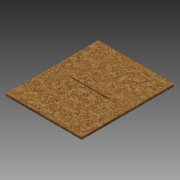
# Autodesk Inventor part: gora
Saved by Autodesk Inventor 2013 (Build 170138000, 138)
## iProperties
Created: 2014-04-26
Part Number: gora
Material: Generic
Document SubType Name: Modeling
Designer: Masta
Density: 1 g/cm^3
Author: Masta
Autodesk Inventor part; units mm, degrees
ref_plane "YZ Plane" through (0, 0, 0) normal (1, 0, 0) x (0, 1, 0)
ref_plane "XZ Plane" through (0, 0, 0) normal (0, 1, 0) x (-1, 0, 0)
ref_plane "XY Plane" through (0, 0, 0) normal (0, 0, 1) x (1, 0, 0)
sketch "Sketch1" plane through (0, 0, 0) normal (0, 0, 1) x (1, 0, 0)
  line L0 (-300, -366) -> (300, -366)
  line L1 (300, -366) -> (300, 366)
  line L2 (300, 366) -> (-300, 366)
  line L3 (-300, 366) -> (-300, -366)
  line L4 (-300, -366) -> (300, 366) construction
  line L5 (300, -366) -> (-300, 366) construction
  line L6 (150, 10) -> (-150, 10)
  line L7 (-150, 10) -> (-150, 0)
  line L8 (-150, 0) -> (150, 0)
  line L9 (150, 0) -> (150, 10)
  line L10 (150, 10) -> (-150, 0) construction
  line L11 (-150, 10) -> (150, 0) construction
  line L12 (0, 0) -> (0, 5) construction
  dimension "d0" = 600
  dimension "d1" = 732
  dimension "d4" = 300
  dimension "d5" = 10
  dimension "d6" = 5
  constraints: 26 end point, 5 parallel, 4 midpoint, 2 horizontal, 2 perpendicular
  measures "d0" distance of L2.end L1.end
  measures "d1" distance of L1.end L0.end
  measures "d4" distance of L8.end L7.end
  measures "d5" distance of L7.end L6.end
  measures "d6" distance of L12.start L12.end
extrude "Extrusion1" add sketch "Sketch1" along normal blind 18
body "Solid1"
